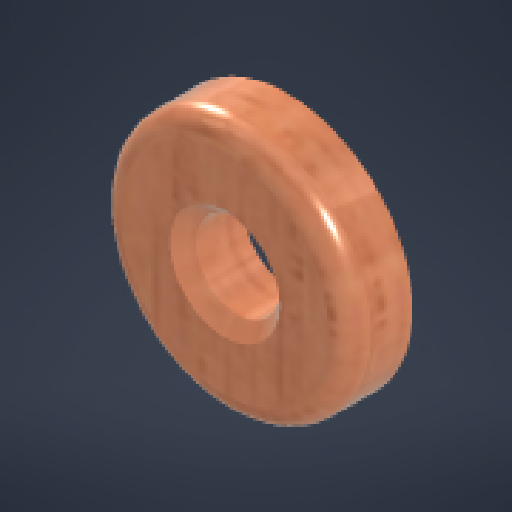
# Autodesk Inventor part: PIVOT_SPACERS,TREBUCHET
Saved by Autodesk Inventor 2026.2 (Build 302298010, 298A)
## iProperties
Created: 2026-02-17
Part Number: PIVOT_SPACERS,TREBUCHET
Material: Wood (Oak)
Document SubType Name: Modeling
Designer: 4aida
Density: 0.76 g/cm^3
Appearance: White Oak - Natural Medium Gloss
Author: 4aida
Autodesk Inventor part; units mm, degrees
ref_plane "YZ Plane" through (0, 0, 0) normal (1, 0, 0) x (0, 1, 0)
ref_plane "XZ Plane" through (0, 0, 0) normal (0, 1, 0) x (-1, 0, 0)
ref_plane "XY Plane" through (0, 0, 0) normal (0, 0, 1) x (1, 0, 0)
sketch "Sketch1" plane through (0, 0, 0) normal (0, 0, 1) x (1, 0, 0)
  circle A0 centre (0, 0) radius 19.05
  circle A1 centre (0, 0) radius 6.35
  point P0 (0, -19.05)
  point P1 (0, 19.05)
  dimension "d0" = 38.1
  dimension "d1" = 12.7
  constraints: 2 centre point, 2 coincident, 2 vertical alignment
  measures "d0" diameter of A0
  measures "d1" diameter of A1
extrude "Extrusion1" add sketch "Sketch1" along normal blind 9.525
chamfer "Chamfer1" distance 2 angle 45 1 edges at (-6.35, 0, 9.525)
fillet "Fillet2" radius 3.175 1 edges at (-19.05, 0, 9.525)
body "Solid1"
